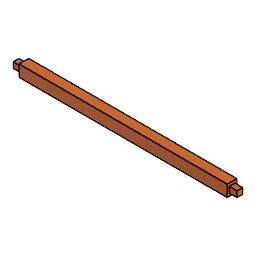
stretcher (Autodesk Fusion 360 design; units mm, degrees)
part number: 2026-08-18-19-37-08-848
Autodesk Fusion 360 part; units mm, degrees
sketch "Sketch1" plane through (0, 0, 0) normal (0, 0, 1) x (1, 0, 0)
  line L0 (0, 0) -> (214, 0)
  line L1 (214, 0) -> (214, 10)
  line L2 (214, 10) -> (0, 10)
  line L3 (0, 10) -> (0, 0)
extrude "Extrude1" add sketch "Sketch1" along normal blind 12 makes body 1
sketch "Sketch2" plane through (0, 0, 0) normal (0, 0, 1) x (1, 0, 0)
  line L0 (-8, 2) -> (0, 2)
  line L1 (0, 2) -> (0, 8)
  line L2 (0, 8) -> (-8, 8)
  line L3 (-8, 8) -> (-8, 2)
extrude "Extrude2" add sketch "Sketch2" along normal blind 6 from surface at 3 separate body makes body 2
sketch "Sketch3" plane through (0, 0, 0) normal (0, 0, 1) x (1, 0, 0)
  line L0 (214, 2) -> (222, 2)
  line L1 (222, 2) -> (222, 8)
  line L2 (222, 8) -> (214, 8)
  line L3 (214, 8) -> (214, 2)
extrude "Extrude3" add sketch "Sketch3" along normal blind 6 from surface at 3 separate body makes body 3
combine "Combine1" operation add target body 1 tool bodies 2 3
named bodies: "Тело"
